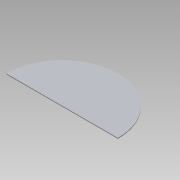
# Autodesk Inventor part: Juring Setengah Lingkaran
Saved by Autodesk Inventor 2015 SP1 (Build 190203100, 203)
## iProperties
Created: 2015-01-29
Part Number: Juring Setengah Lingkaran
Material: Generic
Document SubType Name: Modeling
Designer: Rafi Kurnia Putra
Density: 1 g/cm^3
Appearance: White
Author: Rafi Kurnia Putra
Autodesk Inventor part; units mm, degrees
ref_plane "YZ Plane" through (0, 0, 0) normal (1, 0, 0) x (0, 1, 0)
ref_plane "XZ Plane" through (0, 0, 0) normal (0, 1, 0) x (-1, 0, 0)
ref_plane "XY Plane" through (0, 0, 0) normal (0, 0, 1) x (1, 0, 0)
sketch "Sketch1" plane through (0, 0, 0) normal (0, 1, 0) x (-1, 0, 0)
  arc A0 (-300, 0) -> (300, 0) centre (0, 0) ccw
  line L0 (0, 0) -> (-300, 0)
  line L1 (0, 0) -> (300, 0)
  dimension "d0" = 300
  dimension "d1" = 180
  constraints: 4 end point, 2 point on circle, 1 centre point, 1 coincident
  measures "d0" radius of A0
  measures "d1" angle of L0 L1
extrude "Extrusion1" add sketch "Sketch1" along normal blind 4
body "Solid1"
